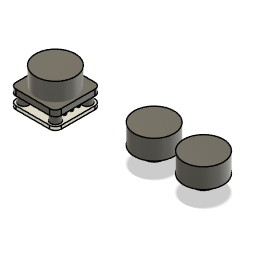
TestSensoriHallCoppette v7 (Autodesk Fusion 360 archive; units mm, degrees)
design "AS5600_test_jig"
Autodesk Fusion 360 part; units mm, degrees
sketch "Sketch2" plane through (0, 0, 0) normal (0, 1, 0) x (1, 0, 0)
  line L0 (-8.5, -11.5) -> (8.5, -11.5)
  line L1 (11.5, -8.5) -> (11.5, 8.5)
  line L2 (8.5, 11.5) -> (-8.5, 11.5)
  line L3 (-11.5, 8.5) -> (-11.5, -8.5)
  line L4 (-11.5, -11.5) -> (11.5, 11.5) construction
  line L5 (11.5, -11.5) -> (-11.5, 11.5) construction
  line L6 (-8, 8) -> (8, 8) construction
  line L7 (8, 8) -> (8, -8) construction
  line L8 (8, -8) -> (-8, -8) construction
  line L9 (-8, -8) -> (-8, 8) construction
  line L10 (-8, 8) -> (8, -8) construction
  line L11 (8, 8) -> (-8, -8) construction
  circle A0 centre (-8, 8) radius 1.7
  circle A1 centre (8, 8) radius 1.7
  circle A2 centre (8, -8) radius 1.7
  circle A3 centre (-8, -8) radius 1.7
  arc A4 (-8.5, 11.5) -> (-11.5, 8.5) centre (-8.5, 8.5) ccw
  arc A5 (11.5, 8.5) -> (8.5, 11.5) centre (8.5, 8.5) ccw
  arc A6 (8.5, -11.5) -> (11.5, -8.5) centre (8.5, -8.5) ccw
  arc A7 (-11.5, -8.5) -> (-8.5, -11.5) centre (-8.5, -8.5) ccw
  line L12 (-2.5, -2.1) -> (2.5, -2.1)
  line L13 (2.5, -2.1) -> (2.5, 2.1)
  line L14 (2.5, 2.1) -> (-2.5, 2.1)
  line L15 (-2.5, 2.1) -> (-2.5, -2.1)
  line L16 (-2.5, -2.1) -> (2.5, 2.1) construction
  line L17 (2.5, -2.1) -> (-2.5, 2.1) construction
  circle A8 centre (-4.12, 6.5) radius 0.5
  circle A9 centre (-1.58, 6.5) radius 0.5
  circle A10 centre (0.96, 6.5) radius 0.5
  circle A11 centre (3.5, 6.5) radius 0.5
  line L18 (-4.12, 6.5) -> (-1.58, 6.5) construction
  line L19 (-1.58, 6.5) -> (0.96, 6.5) construction
  line L20 (0.96, 6.5) -> (3.5, 6.5) construction
  circle A12 centre (2.14, -6.5) radius 0.5
  circle A13 centre (-0.4, -6.5) radius 0.5
  circle A14 centre (-2.94, -6.5) radius 0.5
  line L21 (-2.94, -6.5) -> (-0.4, -6.5) construction
  line L22 (-0.4, -6.5) -> (2.14, -6.5) construction
  line L23 (-6.9, 3.63) -> (-5.02, 3.63)
  line L24 (-5.02, 3.63) -> (-5.02, 2.63)
  line L25 (-5.02, 2.63) -> (-6.9, 2.63)
  line L26 (-6.9, 2.63) -> (-6.9, 3.63)
  line L27 (-6.9, 0.63) -> (-5.02, 0.63)
  line L28 (-5.02, 0.63) -> (-5.02, -0.37)
  line L29 (-5.02, -0.37) -> (-6.9, -0.37)
  line L30 (-6.9, -0.37) -> (-6.9, 0.63)
  line L31 (-6.9, -2.37) -> (-5.02, -2.37)
  line L32 (-5.02, -2.37) -> (-5.02, -3.37)
  line L33 (-5.02, -3.37) -> (-6.9, -3.37)
  line L34 (-6.9, -3.37) -> (-6.9, -2.37)
  line L35 (-6.9, 2.63) -> (-6.9, 0.63) construction
  line L36 (-6.9, -0.37) -> (-6.9, -2.37) construction
  line L37 (6.22, 4.5) -> (8.1, 4.5)
  line L38 (8.1, 4.5) -> (8.1, 3.5)
  line L39 (8.1, 3.5) -> (6.22, 3.5)
  line L40 (6.22, 3.5) -> (6.22, 4.5)
  line L41 (6.22, 1) -> (8.1, 1)
  line L42 (8.1, 1) -> (8.1, 0)
  line L43 (8.1, 0) -> (6.22, 0)
  line L44 (6.22, 0) -> (6.22, 1)
  line L45 (6.22, -2.5) -> (8.1, -2.5)
  line L46 (8.1, -2.5) -> (8.1, -3.5)
  line L47 (8.1, -3.5) -> (6.22, -3.5)
  line L48 (6.22, -3.5) -> (6.22, -2.5)
  line L49 (8.1, -2.5) -> (8.1, 0) construction
  line L50 (8.1, 3.5) -> (8.1, 1) construction
  circle A15 centre (8, -8) radius 2.5
  circle A16 centre (8, 8) radius 2.5
  circle A17 centre (-8, 8) radius 2.5
  circle A18 centre (-8, -8) radius 2.5
  dimension "d6" = 23
  dimension "d7" = 23
  dimension "d8" = 16
  dimension "d9" = 16
  dimension "d10" = 3.4
  dimension "d11" = 3
  dimension "d12" = 3
  dimension "d13" = 3
  dimension "d14" = 3
  dimension "d15" = 5
  dimension "d16" = 4.2
  dimension "d21" = 1
  dimension "d25" = 2.54
  dimension "d26" = 2.54
  dimension "d27" = 2.54
  dimension "d28" = 5
  dimension "d29" = 8
  dimension "d30" = 2.54
  dimension "d31" = 2.54
  dimension "d32" = 5
  dimension "d33" = 8.56
  dimension "d34" = 1.88
  dimension "d35" = 1
  dimension "d36" = 2
  dimension "d37" = 2
  dimension "d38" = 4.6
  dimension "d39" = 8.13
  dimension "d41" = 3.4
  dimension "d42" = 2.5
  dimension "d43" = 2.5
  dimension "d44" = 8
  dimension "d49" = 5
  dimension "d51" = 360
  constraint horizontal L0
  constraint perpendicular L0 L1
  constraint parallel L0 L2
  constraint parallel L1 L3
  constraint coincident L4 origin
  constraint coincident L5 origin
  constraint horizontal L6
  constraint perpendicular L6 L7
  constraint parallel L6 L8
  constraint parallel L7 L9
  constraint coincident L10 origin
  constraint coincident L11 origin
  constraint coincident L6.start L9.end
  constraint coincident L6.end L7.start
  constraint coincident L7.end L8.start
  constraint coincident L8.end L9.start
  constraint equal A0 A3
  constraint equal A1 A3
  constraint equal A2 A3
  constraint coincident L5.end L3
  constraint coincident L5.end L2
  constraint tangent L3 A4
  constraint tangent L2 A4
  constraint coincident L4.end L2
  constraint coincident L4.end L1
  constraint tangent L2 A5
  constraint tangent L1 A5
  constraint coincident L5.start L0
  constraint coincident L5.start L1
  constraint tangent L0 A6
  constraint tangent L1 A6
  constraint coincident L4.start L3
  constraint coincident L4.start L0
  constraint tangent L3 A7
  constraint tangent L0 A7
  constraint horizontal L12
  constraint perpendicular L12 L13
  constraint parallel L12 L14
  constraint parallel L13 L15
  constraint coincident L16 origin
  constraint coincident L17 origin
  constraint coincident A8.centre L18.start
  constraint coincident A9.centre L18.end
  constraint parallel L6 L18
  constraint coincident A10.centre L19.end
  constraint coincident A11.centre L20.end
  constraint horizontal L19
  constraint horizontal L20
  constraint equal A8 A9
  constraint equal A8 A10
  constraint equal A8 A11
  constraint equal A8 A14
  constraint equal A9 A13
  constraint equal A10 A12
  constraint coincident A14.centre L21.start
  constraint coincident A13.centre L21.end
  constraint horizontal L21
  constraint coincident A12.centre L22.end
  constraint horizontal L22
  constraint horizontal L23
  constraint vertical L24
  constraint horizontal L25
  constraint vertical L26
  constraint horizontal L27
  constraint vertical L28
  constraint horizontal L29
  constraint vertical L30
  constraint horizontal L31
  constraint vertical L32
  constraint horizontal L33
  constraint vertical L34
  constraint equal L23 L27
  constraint equal L27 L31
  constraint equal L24 L28
  constraint equal L28 L32
  constraint vertical L35
  constraint vertical L36
  constraint horizontal L37
  constraint vertical L38
  constraint horizontal L39
  constraint vertical L40
  constraint horizontal L41
  constraint vertical L42
  constraint horizontal L43
  constraint vertical L44
  constraint horizontal L45
  constraint vertical L46
  constraint horizontal L47
  constraint vertical L48
  constraint equal L23 L37
  constraint equal L24 L38
  constraint equal L23 L41
  constraint equal L24 L42
  constraint equal L23 L45
  constraint equal L24 L48
  constraint vertical L50
  constraint vertical L49
  constraint concentric A2 A15
  measures "d6" distance of L4.start L5.start
  measures "d7" distance of L5.start L4.end
  measures "d8" distance of L7.end L8.end
  measures "d9" distance of L6.end L7.end
  measures "d10" diameter of A3
  measures "d11" radius of A4
  measures "d12" radius of A5
  measures "d13" radius of A6
  measures "d14" radius of A7
  measures "d15" distance of L13.end L14.end
  measures "d16" distance of L12.end L13.end
  measures "d21" diameter of A8
  measures "d25" distance of A8.centre A9.centre
  measures "d26" horizontal distance of A9.centre A10.centre
  measures "d27" horizontal distance of A10.centre A11.centre
  measures "d28" distance of L2 L18
  measures "d29" distance of L1 A11.centre
  measures "d30" distance of A13.centre A14.centre
  measures "d31" horizontal distance of A12.centre A13.centre
  measures "d32" distance of L0 L22
  measures "d33" distance of L3 A14.centre
  measures "d34" distance of L23.start L23.end
  measures "d35" distance of L23.end L24.end
  measures "d36" distance of L25 L27
  measures "d37" distance of L29 L31
  measures "d38" distance of L3 L35
  measures "d39" distance of L0 L33
  measures "d41" distance of L1 L50
  measures "d42" distance of L38.end L41.end
  measures "d43" distance of L42.end L45.end
  measures "d44" distance of L0 L47
  measures "d49" diameter of A15
extrude "Extrude1" add sketch "Sketch2" against normal blind 1.7 contours L0 L1 L2 L3 A4 A5 A6 A7 | L12 L13 L14 L15 | L23 L24 L25 L26 | L27 L28 L29 L30 | L31 L32 L33 L34 | L37 L38 L39 L40 | L41 L42 L43 L44 | L45 L46 L47 L48 | A15 | A16 | A17 | A18 makes body 1
extrude "Extrude2" add sketch "Sketch2" along normal blind 1.8 contours L12 L13 L14 L15 bodies 1
extrude "Extrude3" add sketch "Sketch2" along normal blind 0.8 contours L23 L24 L25 L26 | L37 L38 L39 L40 | L41 L42 L43 L44 | L45 L46 L47 L48 bodies 1
extrude "Extrude4" add sketch "Sketch2" along normal blind 1.22 contours L27 L28 L29 L30 | L31 L32 L33 L34 bodies 1
extrude "Estrusione5" add sketch "Sketch2" against normal blind 2 draft -3 separate body contours A0 | A1 | A2 | A3 makes body 2 at (-7.1616, -0.4444, 9.4521) makes body 3 at (9.5107, -0.4444, -7.2725) makes body 4 at (6.9546, -0.4444, 9.3109) makes body 5 at (-7.1616, -0.4444, -6.5479)
sketch "Schizzo3" plane through (0, 1.8, 0) normal (0, 1, 0) x (-1, 0, 0)
  line L0 (2.5, -2.1) -> (2.5, 2.1)
  line L1 (2.5, 2.1) -> (-2.5, 2.1)
  line L2 (-2.5, 2.1) -> (-2.5, -2.1)
  line L3 (-2.5, -2.1) -> (2.5, -2.1)
  circle A0 centre (0, 0) radius 1.5
  dimension "d56" = 3
  constraint coincident A0.centre origin
  measures "d56" diameter of A0
extrude "Estrusione7" add sketch "Schizzo3" along normal blind 0.5 contours A0 bodies 5 1 2 3 4
sketch "Schizzo4" plane through (0, 2.3, 0) normal (0, 1, 0) x (-1, 0, 0)
  circle A0 centre (0, 0) radius 1.5
  circle A1 centre (0, 0) radius 2.05
  dimension "d59" = 4.1
  constraint coincident A0.centre A1.centre
  measures "d59" diameter of A1
extrude "Estrusione8" cut sketch "Schizzo4" against normal blind 0.5 contours A0 bodies 1 4 3 2 5
extrude "Estrusione9" add sketch "Schizzo4" along normal blind 2 separate body contours A0 | A1 makes body 6
sketch "Schizzo5" plane through (0, 4.3, 0) normal (0, 1, 0) x (-1, 0, 0)
  circle A0 centre (0, 0) radius 2.05
  circle A1 centre (0, 0) radius 5
  dimension "d64" = 10
  constraint concentric A0 A1
  measures "d64" diameter of A1
extrude "Estrusione6" add sketch "Sketch2" along normal up to surface (4.3 mm away) separate body contours A0 | A1 | A2 | A3 | A15 | A16 | A17 | A18 makes body 7 at (10.4969, 2.8667, 8.1246) makes body 8 at (-5.5031, 2.8667, 8.1246) makes body 9 at (10.4969, 2.8667, -7.8754) makes body 10 at (-5.5031, 2.8667, -7.8754)
sketch "Schizzo6" plane through (0, 0, 0) normal (0, 1, 0) x (1, 0, 0)
  line L0 (11.5, 11.5, 4.3) -> (-11.5, 11.5, 4.3)
  line L1 (-11.5, 11.5, 4.3) -> (-11.5, -11.5, 4.3)
  line L2 (-11.5, -11.5, 4.3) -> (11.5, -11.5, 4.3)
  line L3 (11.5, -11.5, 4.3) -> (11.5, 11.5, 4.3)
  line L4 (-11.5, 11.5, 4.3) -> (11.5, -11.5, 4.3)
  line L5 (11.5, 11.5, 4.3) -> (-11.5, -11.5, 4.3)
  circle A0 through (5, 0, 4.3) (-2.5, 4.3301, 4.3) (-2.5, -4.3301, 4.3)
  circle A1 through (4.9, 0, 4.3) (-2.45, 4.2435, 4.3) (-2.45, -4.2435, 4.3)
  point P0 (0, 0)
  dimension "d70" = 10
  dimension "d73" = 9.8
extrude "Estrusione10" add sketch "Schizzo6" along normal blind 3 contours L0 L4 L5 A0 | L3 L4 L5 A0 | L1 L4 L5 A0 | L2 L4 L5 A0 | L4 L5 A0 A1 | L4 L5 A0 A1 | L4 L5 A0 A1 | L4 L5 A0 A1 | L4 L5 A1 | L4 L5 A1 | L4 L5 A1 | L4 L5 A1 in plane through (0, 4.3, 0) normal (0, 1, 0) bodies 6 8 7 10 9
fillet "Raccordo1" radius 3 4 edges at (11.5, 5.8, -11.5) (-11.5, 5.8, -11.5) (-11.5, 5.8, 11.5) (11.5, 5.8, 11.5) on bodies 6
extrude "Estrusione11" cut sketch "Schizzo6" along normal blind 2 contours L4 L5 A0 A1 | L4 L5 A0 A1 | L4 L5 A0 A1 | L4 L5 A0 A1 | L4 L5 A1 | L4 L5 A1 | L4 L5 A1 | L4 L5 A1 in plane through (0, 4.3, 0) normal (0, 1, 0) bodies 2 3 4 5 1 6 makes body 11 at (-2.0398, 3.6333, -0.2041)
combine "Combina1" operation add target body 6 tool bodies 2 4 3 5
extrude "Estrusione12" add sketch "Schizzo6" along normal blind 2 separate body contours L4 L5 A1 | L4 L5 A1 | L4 L5 A1 | L4 L5 A1 in plane through (0, 4.3, 0) normal (0, 1, 0) makes body 12
sketch "Schizzo7" plane through (0, 6.3, 0) normal (0, 1, 0) x (-1, 0, 0)
  circle A0 centre (0, 0) radius 4.9
  circle A1 centre (0, 0) radius 10
  constraint coincident A0.centre A1.centre
extrude "Estrusione13" add sketch "Schizzo7" along normal blind 10 separate body contours A0 | A1 makes body 13
combine "Combina2" operation add target body 12 tool bodies 13
sketch "Schizzo8" plane through (0, 4.3, 0) normal (0, -1, 0) x (1, 0, 0)
  circle A0 centre (0, 0) radius 4.9
  circle A1 centre (0, 0) radius 2.2
  dimension "d78" = 4.4
  constraint concentric A0 A1
  measures "d78" diameter of A1
extrude "Estrusione14" add sketch "Schizzo8" along normal blind 2 bodies 12
copy_body "CopiaIncollaCorpi1" bodies 12 makes body 14
move_body "Sposta1" bodies 14 to x (1, 0, 0) y (0, 1, 0) z (0, 0, 1) at (50, 0, 0)
copy_body "CopiaIncollaCorpi2" bodies 12 makes body 15
move_body "Sposta2" bodies 15 to x (1, 0, 0) y (0, 1, 0) z (0, 0, 1) at (75, 0, 0)
copy_body "CopiaIncollaCorpi3" [suppressed]
move_body "Sposta3" [suppressed]
extrude "Estrusione15" [suppressed]
extrude "Estrusione16" [suppressed]
extrude "Estrusione17" [suppressed]
extrude "Estrusione18" [suppressed]
extrude "Estrusione19" [suppressed]
extrude "Estrusione20" [suppressed]
copy_body "CopiaIncollaCorpi5" [suppressed]
move_body "Sposta6" [suppressed]
extrude "Estrusione23" [suppressed]
extrude "Estrusione24" [suppressed]
move_body "Sposta7" [suppressed]
extrude "Estrusione25" [suppressed]
named bodies: "AS5600", "Base", "Magnete", "Rotore0.5", "Rotore2.5", "Rotore0.5 (1)", "Rotore3.5", "Rotore0.5 (2)", "Rotore4.5", "Rotore1.5 (1)", "Rotore1.5"
